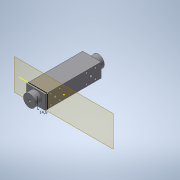
# Autodesk Inventor part: wheel-adapter-rear
Saved by Autodesk Inventor 2020 (Build 240168000, 168)
## iProperties
Created: 2020-05-14
Part Number: wheel-adapter-rear
Material: Ogólny
Document SubType Name: Modeling
Designer: blep
Density: 1 g/cm^3
Appearance: Domyślna
Author: blep
Autodesk Inventor part; units mm, degrees
ref_plane "YZ Plane" through (0, 0, 0) normal (1, 0, 0) x (0, 1, 0)
ref_plane "XZ Plane" through (0, 0, 0) normal (0, 1, 0) x (-1, 0, 0)
ref_plane "Płaszczyzna konstrukcyjna1" through (0, 0, 0) normal (0, 0, 1) x (1, 0, 0)
sketch "Szkic1" plane through (0, 0, 0) normal (0, 0, 1) x (1, 0, 0)
  line L0 (-70.3592, -33) -> (-26.3592, -33)
  line L1 (-26.3592, -33) -> (-26.3592, -11)
  line L2 (-26.3592, -11) -> (-70.3592, -11)
  line L3 (-70.3592, -11) -> (-70.3592, -33)
  line L4 (-70.3592, -11) -> (-26.3592, -11) projected
  line L5 (-26.3592, -11) -> (-26.3592, -33) projected
  point P0 (0, 0)
  constraints: 8 end point, 4 collinear, 2 parallel, 1 horizontal, 1 perpendicular
extrude "Wyciągnięcie proste1" add sketch "Szkic1" against normal blind 3
sketch "Szkic2" plane through (0, 0, -3) normal (0, 0, -1) x (-1, 0, 0)
  line L0 (32.3592, -11) -> (26.3592, -11)
  line L1 (26.3592, -11) -> (26.3592, -33)
  line L2 (26.3592, -33) -> (32.3592, -33)
  line L3 (32.3592, -33) -> (32.3592, -11)
  line L4 (26.3592, -11) -> (26.3592, -33) projected
  line L5 (26.3592, -33) -> (70.3592, -33) projected
  line L6 (70.3592, -11) -> (26.3592, -11) projected
  point P0 (0, 0)
  dimension "d2" = 6
  constraints: 8 end point, 3 collinear, 2 parallel, 1 horizontal, 1 perpendicular
  measures "d2" distance between parallel lines of L1 L3
extrude "Wyciągnięcie proste2" add sketch "Szkic2" along normal blind 20
sketch "Szkic3" plane through (-26.3592, -33, 0) normal (1, 0, 0) x (0, 0, -1)
  circle A0 centre (6, 3.3) radius 1.25 projected
  circle A1 centre (20, 3.3) radius 1.25 projected
  circle A2 centre (20, 18.7) radius 1.25 projected
  circle A3 centre (6, 18.7) radius 1.25 projected
  circle A4 centre (20, 3.3) radius 1.5
  circle A5 centre (6, 3.3) radius 1.5
  circle A6 centre (20, 18.7) radius 1.5
  circle A7 centre (6, 18.7) radius 1.5
  circle A8 centre (13, 11) radius 2.125 projected
  point P0 (0, 33)
  dimension "d5" = 0.25
  dimension "d6" = 0.25
  dimension "d7" = 0.25
  dimension "d8" = 0.25
  constraints: 4 centre point
  measures "d5" radial gap between concentric circles of A1 A4
  measures "d6" radial gap between concentric circles of A0 A5
  measures "d7" radial gap between concentric circles of A2 A6
  measures "d8" radial gap between concentric circles of A3 A7
extrude "Wyciągnięcie proste3" cut sketch "Szkic3" against normal through all contours A0 | A1 | A2 | A3 | A4 | A5 | A6 | A7 | A8
sketch "Szkic4" plane through (0, 0, 0) normal (0, 0, 1) x (1, 0, 0)
  line L0 (-40.9592, -22) -> (-40.9592, -11) construction
  line L1 (-70.3592, -11) -> (-32.3592, -11) construction
  line L2 (-40.9592, -22) -> (-40.9592, -33) construction
  line L3 (-70.3592, -33) -> (-26.3592, -33) construction
  line L4 (-26.3592, -33) -> (-26.3592, -11) construction
  line L5 (-55.5592, -11) -> (-26.3592, -11)
  line L6 (-26.3592, -11) -> (-26.3592, -33)
  line L7 (-26.3592, -33) -> (-55.5592, -33)
  line L8 (-55.5592, -33) -> (-55.5592, -11)
  line L9 (-40.9592, -22) -> (-55.5592, -22) construction
  line L10 (-40.9592, -22) -> (-26.3592, -22) construction
  line L11 (-26.3592, -11) -> (-70.3592, -11) projected
  point P0 (0, 0)
  dimension "d11" = 14.6
  constraints: 16 end point, 4 collinear, 3 horizontal, 2 midpoint, 2 parallel, 2 perpendicular, 2 point on line, 1 vertical
  measures "d11" distance from line of L4 L0.start
extrude "Wyciągnięcie proste4" cut sketch "Szkic4" against normal through all keep common part
ref_plane "Płaszczyzna konstrukcyjna2" through (-49.4592, -8.3, 3) normal (0, 0, 1) x (1, 0, 0)
sketch "Szkic5" plane through (0, 0, 0) normal (0, 0, 1) x (1, 0, 0)
  line L0 (-55.5592, -33) -> (-55.5592, -11) projected
  line L1 (-55.5592, -33) -> (-26.3592, -33) projected
  line L2 (-26.3592, -33) -> (-26.3592, -11) projected
  line L3 (-26.3592, -11) -> (-55.5592, -11) projected
  point P0 (0, 0)
extrude "Wyciągnięcie proste5" add sketch "Szkic5" along normal blind 3
hole "Otwór3" at (-40.9592, -22, 0) direction (0, 0, -1) diameter 4.25 end through all both
sketch "Szkic7" plane through (0, 0, 3) normal (0, 0, 1) x (1, 0, 0)
  circle A0 centre (-40.9592, -22) radius 10 projected
  circle A1 centre (-40.9592, -22) radius 2.125 projected
  circle A2 centre (-40.9592, -22) radius 10 projected
  circle A3 centre (-40.9592, -22) radius 9.5
  point P0 (0, 0)
  dimension "d42" = 0.5
  constraints: 1 centre point
  measures "d42" radial gap between concentric circles of A0 A3
extrude "Wyciągnięcie proste8" add sketch "Szkic7" along normal blind 10 contours A3
sketch "Szkic6" plane through (0, 0, -3) normal (0, 0, -1) x (-1, 0, 0)
  circle A0 centre (40.9592, -22) radius 2.125 projected
  circle A1 centre (40.9592, -22) radius 4.5
  point P0 (0, 0)
  dimension "d37" = 9
  constraints: 1 centre point, 1 coincident
  measures "d37" diameter of A1
extrude "Wyciągnięcie proste7" cut sketch "Szkic6" against normal blind 12 contours A0 | A1
sketch "Szkic8" plane through (0, 0, -23) normal (0, 0, -1) x (-1, 0, 0)
  line L0 (26.3592, -33) -> (32.3592, -33) projected
  line L1 (32.3592, -33) -> (32.3592, -11) projected
  line L2 (32.3592, -11) -> (26.3592, -11) projected
  line L3 (26.3592, -11) -> (26.3592, -33) projected
  point P0 (0, 0)
extrude "Wyciągnięcie proste9" add sketch "Szkic8" along normal blind 18
mirror "Odbij1" about plane through (-29.3592, -22, -41) normal (0, 0, -1)
sketch "Szkic9" plane through (-32.3592, -33, -3) normal (-1, 0, 0) x (0, 0, 1)
  circle A0 centre (-66, 11) radius 2.125 projected
  circle A1 centre (-59, 18.7) radius 1.5 projected
  circle A2 centre (-59, 3.3) radius 1.5 projected
  circle A3 centre (-73, 18.7) radius 1.5 projected
  circle A4 centre (-73, 3.3) radius 1.5 projected
  circle A5 centre (-3, 3.3) radius 1.5 projected
  circle A6 centre (-3, 18.7) radius 1.5 projected
  circle A7 centre (-17, 3.3) radius 1.5 projected
  circle A8 centre (-17, 18.7) radius 1.5 projected
  circle A9 centre (-10, 11) radius 2.125 projected
  line L0 (0, 22) -> (0, 0) projected
  line L1 (0, 22) -> (-76, 22) projected
  line L2 (-76, 22) -> (-76, 0) projected
  line L3 (0, 0) -> (-76, 0) projected
  circle A10 centre (-66, 11) radius 2.125 projected
  circle A11 centre (-66, 11) radius 4.5
  circle A12 centre (-10, 11) radius 2.125 projected
  circle A13 centre (-10, 11) radius 4.5
  point P0 (3, 33)
  dimension "d47" = 9
  dimension "d48" = 9
  constraints: 2 centre point, 2 coincident
  measures "d47" diameter of A11
  measures "d48" diameter of A13
extrude "Wyciągnięcie proste10" add sketch "Szkic9" along normal up to surface (23.2 mm away) contours L0 L3 L2 L1
sketch "Szkic11" plane through (-55.5592, -33, 3) normal (-1, 0, 0) x (0, 0, 1)
  line L0 (-86, 15.5) -> (-67.5, 15.5)
  line L1 (-67.5, 15.5) -> (-67.5, 6.5)
  line L2 (-67.5, 6.5) -> (-86, 6.5)
  line L3 (-86, 6.5) -> (-86, 15.5)
  line L4 (-20.5, 15.5) -> (-2, 15.5)
  line L5 (-2, 15.5) -> (-2, 6.5)
  line L6 (-2, 6.5) -> (-20.5, 6.5)
  line L7 (-20.5, 6.5) -> (-20.5, 15.5)
  line L8 (0, 22) -> (0, 0) projected
  line L9 (-88, 22) -> (-88, 0) projected
  circle A0 centre (-72, 11) radius 4.5 projected
  circle A1 centre (-16, 11) radius 4.5 projected
  point P0 (-3, 33)
  dimension "d51" = 2
  dimension "d53" = 2
  constraints: 16 end point, 4 parallel, 4 tangent, 2 collinear, 2 horizontal, 2 perpendicular
  measures "d51" distance between parallel lines of L8 L5
  measures "d53" distance between parallel lines of L9 L3
extrude "Wyciągnięcie proste11" cut sketch "Szkic11" against normal blind 19.1
equation "\"d53\" = d51"
